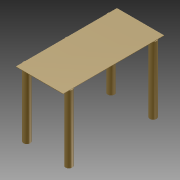
# Autodesk Inventor part: G1P-trmnls
Saved by Autodesk Inventor 2011 SP1 (Build 150282100, 282)
## iProperties
Created: 2013-12-24
Part Number: G1P-trmnls
Catalog Web Link: www.cadenas.de
Description: G Series - Process Sealed Ultra-Miniature Toggles -terrminals-
Vendor: NKKSWITCHES
Document SubType Name: Modeling
Designer: PARTuser1
Manufacturer: NKKSWITCHES
Density: 1 g/cm^3
Category: PARTsolutions
Company: NKKSWITCHES
Title: G1P-trmnls
Author: Cadenas PARTsolutions
PSOL_IDENT_0: {$CADENAS_DATA\23d-libs\nkkswitches\toggle\g\parts\g_terminals.prj},227 {VTYP=3D},{NB=G1P-trmnls},{L
PSOL_IDENT_1: INA=G1P-trmnls},{NN=G Series - Process Sealed Ultra-Miniature Toggles -terrminals},{DATE=23.03.2009
PSOL_IDENT_2: 07:46:36},{GEOMDATE=12.03.2009 00:00:00},{VERSION=},{LINEID=10},{LINESUBID=-1},{WBVAR=PLS,TRMNLS}  {
PSOL_IDENT_3: NB=G1P-trmnls},{LINA=G1P-trmnls},{KT=DUMMY},{PN=G1P},{SRS=G},{PLS=1},{TRMNLS=P}
CNS_NN: G Series - Process Sealed Ultra-Miniature Toggles -terrminals
CNS_NB: G1P-trmnls
CNS_NBSYN: $PN.-trmnls
CNS_LINA: G1P-trmnls
CNS_PN: G1P
CNS_SRS: G
CNS_PLS: 1 - SPDT
CNS_TRMNLS: P - Straight
SUPPLIER: NKKSWITCHES
ARTICLENO: G1P-trmnls
BOMINFO: G1P-trmnls
CREATOR: CADENAS GmbH
Autodesk Inventor part; units mm, degrees
ref_plane "YZ Plane" through (0, 0, 0) normal (1, 0, 0) x (0, 1, 0)
ref_plane "XZ Plane" through (0, 0, 0) normal (0, 1, 0) x (-1, 0, 0)
ref_plane "XY Plane" through (0, 0, 0) normal (0, 0, 1) x (1, 0, 0)
sketch "Sketch_1" plane through (0, 0, 0) normal (0, 1, 0) x (-1, 0, 0)
  line L0 (1.4224, 3.048) -> (-1.4224, 3.048)
  line L1 (-1.4224, 3.048) -> (-1.4224, -3.048)
  line L2 (-1.4224, -3.048) -> (1.4224, -3.048)
  line L3 (1.4224, -3.048) -> (1.4224, 3.048)
  constraints: 8 end point
extrude "Extrusion1" add sketch "Sketch_1" along normal blind 0.0254
sketch "Sketch_2" plane through (0, 0, 0) normal (0, 1, 0) x (-1, 0, 0)
  circle A0 centre (-1.27, -2.54) radius 0.2032
  constraints: 1 centre point
extrude "Extrusion2" add sketch "Sketch_2" against normal blind 4.064
pattern_linear "Rectangular Pattern1" count 2 spacing 2.54 along (-1, 0, 0) count 3 spacing 2.54 along (0, 0, 1) of "Extrusion2" skipped copies 2
ref_plane "to_body_XY" through (0, -0.508, 0) normal (0, -1, 0) x (1, 0, 0)
ref_plane "to_body_YZ" through (0, -0.508, 0) normal (1, 0, 0) x (0, 0, 1)
ref_plane "to_body_ZX" through (0, -0.508, 0) normal (0, 0, 1) x (0, -1, 0)
body "Solid1"
